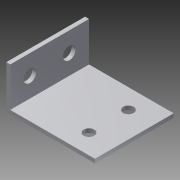
# Autodesk Inventor part: 爪_根本
Saved by Autodesk Inventor 2015 (Build 190159000, 159)
## iProperties
Created: 2015-05-18
Part Number: 爪_根本
Material: アルミニウム 1100-H14
Document SubType Name: Modeling
Designer: kenta
Density: 2.7 g/cm^3
Appearance: サテン
Mass: 1.68065 g
Surface Area: 13.87 cm^2
Volume: 0.622464 cm^3
Author: kenta
Autodesk Inventor part; units mm, degrees
ref_plane "YZ Plane" through (0, 0, 0) normal (1, 0, 0) x (0, 1, 0)
ref_plane "XZ Plane" through (0, 0, 0) normal (0, 1, 0) x (-1, 0, 0)
ref_plane "XY Plane" through (0, 0, 0) normal (0, 0, 1) x (1, 0, 0)
sketch "スケッチ3" plane through (0, 0, 0) normal (0, 0, 1) x (1, 0, 0)
  line L0 (-11.25, 10) -> (11.25, 10)
  line L1 (11.25, 10) -> (11.25, -10)
  line L2 (11.25, -10) -> (-11.25, -10)
  line L3 (-11.25, -10) -> (-11.25, 10)
  line L4 (-11.25, 10) -> (11.25, -10) construction
  line L5 (11.25, 10) -> (-11.25, -10) construction
  point P0 (0, 0)
  dimension "d15" = 22.5
  dimension "d16" = 20
  constraints: 12 end point, 2 midpoint, 2 parallel, 1 horizontal, 1 perpendicular
  measures "d15" distance of L1.end L2.end
  measures "d16" distance of L0.end L1.end
extrude "押し出し2" add sketch "スケッチ3" along normal blind 1
sketch "スケッチ4" plane through (0, 0, 1) normal (0, 0, 1) x (1, 0, 0)
  line L0 (-11.25, 10) -> (-11.25, -10) projected
  line L1 (11.25, 10) -> (-11.25, 10) projected
  line L2 (-11.25, -10) -> (11.25, -10) projected
  point P0 (0, 0)
  point P1 (4.75, 5)
  point P2 (4.75, -5)
  dimension "d19" = 16
  dimension "d20" = 5
  dimension "d21" = 5
  constraints: 1 vertical alignment
  measures "d19" distance from line of L0 point (4.75, 5)
  measures "d20" distance from line of point (4.75, 5) L1
  measures "d21" distance from line of L2 point (4.75, -5)
hole "穴2" at (4.75, 5, 1) at (4.75, -5, 1) direction (0, 0, -1) diameter 2.7 end through all
sketch "スケッチ5" plane through (0, 0, 1) normal (0, 0, 1) x (1, 0, 0)
  line L0 (11.25, -10) -> (-11.25, -10) projected
  line L1 (-11.25, 10) -> (-10.25, 10)
  line L2 (-10.25, 10) -> (-10.25, -10)
  line L3 (-10.25, -10) -> (-11.25, -10)
  line L4 (-11.25, -10) -> (-11.25, 10)
  point P0 (0, 0)
  dimension "d29" = 1
  constraints: 8 end point, 2 parallel, 1 horizontal, 1 perpendicular, 1 point on line
  measures "d29" distance of L2.end L3.end
extrude "押し出し3" add sketch "スケッチ5" along normal blind 10
sketch "スケッチ6" plane through (-10.25, -10, 1) normal (1, 0, 0) x (0, 0, -1)
  line L0 (-10, 0) -> (-10, 20) projected
  line L1 (0, 20) -> (-10, 20) projected
  line L2 (0, 0) -> (-10, 0) projected
  point P0 (1, 10)
  point P1 (-5, 15)
  point P2 (-5, 5)
  dimension "d32" = 5
  dimension "d33" = 5
  dimension "d34" = 5
  constraints: 1 vertical alignment
  measures "d32" distance from line of L0 point (-5, 15)
  measures "d33" distance from line of point (-5, 15) L1
  measures "d34" distance from line of L2 point (-5, 5)
hole "穴3" at (-10.25, 5, 6) at (-10.25, -5, 6) direction (-1, 0, 0) diameter 3.2 end through all
